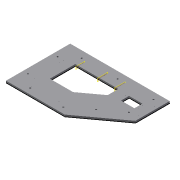
# Autodesk Inventor part: plate
Saved by Autodesk Inventor 2022 (Build 260148000, 148)
## iProperties
Created: 2006-05-17
Part Number: plate
Document SubType Name: Modeling
Designer: dchu
Density: 1 g/cm^3
Material: Generic
Appearance: Default
Author: dchu
Autodesk Inventor part; units mm, degrees
ref_plane "YZ Plane" through (0, 0, 0) normal (1, 0, 0) x (0, 1, 0)
ref_plane "XZ Plane" through (0, 0, 0) normal (0, 1, 0) x (-1, 0, 0)
ref_plane "XY Plane" through (0, 0, 0) normal (0, 0, 1) x (1, 0, 0)
sketch "Sketch1" plane through (0, 0, 0) normal (0, 0, 1) x (1, 0, 0)
  line L0 (1080.9387, 856.8456) -> (-31.0901, 856.8456)
  line L1 (-31.0901, 856.8456) -> (-31.0901, 139.4979)
  line L2 (-31.0901, 139.4979) -> (626.2703, 139.4979)
  line L3 (626.2703, 139.4979) -> (1080.9387, 473.3358)
  line L4 (1080.9387, 473.3358) -> (1080.9387, 856.8456)
  line L5 (963.1788, 520.0847) -> (751.3683, 364.564) construction
  line L6 (195.0188, 687.1378) -> (677.0148, 687.1378)
  line L7 (677.0148, 687.1378) -> (677.0148, 567.5728)
  line L8 (677.0148, 567.5728) -> (453.8217, 403.6944)
  line L9 (453.8217, 403.6944) -> (195.0188, 403.6944)
  line L10 (195.0188, 403.6944) -> (195.0188, 687.1378)
  line L11 (804.0525, 679.6649) -> (953.5087, 679.6649)
  line L12 (953.5087, 679.6649) -> (953.5087, 589.9913)
  line L13 (953.5087, 589.9913) -> (804.0525, 589.9913)
  line L14 (804.0525, 589.9913) -> (804.0525, 679.6649)
  point P0 (175.6092, 779.9153)
  point P1 (575.6092, 779.9153)
  point P2 (975.6092, 781.6554)
  point P3 (545.6092, 203.1178)
  point P4 (175.6092, 203.1178)
  point P5 (25, 660.086)
  point P6 (25, 328.8534)
  dimension "d1" = 400
  dimension "d2" = 400
  dimension "d3" = 370
  constraints: 30 end point, 8 parallel, 4 perpendicular, 2 horizontal, 2 horizontal alignment, 2 vertical alignment
  measures "d1" distance of point (575.609, 779.915) point (175.609, 779.915)
  measures "d2" horizontal distance of point (975.609, 781.655) point (575.609, 779.915)
  measures "d3" distance of point (545.609, 203.118) point (175.609, 203.118)
extrude "Extrusion1" add sketch "Sketch1" along normal blind 20
sketch "Sketch2" plane through (0, 0, 20) normal (0, 0, 1) x (1, 0, 0)
  point P0 (784.2966, 660.4305)
  point P1 (784.2966, 613.0548)
  point P2 (971.9413, 613.0548)
  point P3 (971.9413, 660.4305)
  point P4 (93.4007, 660.4305)
  point P5 (93.4007, 613.0548)
  point P6 (470.1501, 736.9158)
  point P7 (1046.3575, 723.9381)
  point P8 (1046.3575, 539.6556)
  point P9 (470.1501, 230.7876)
  point P10 (163.8777, 230.7876)
  point P11 (106.776, 316.4401)
  point P12 (656.459, 728.2437)
  point P13 (231.1299, 728.2437)
hole "Hole1" at (784.2966, 660.4305, 20) at (784.2966, 613.0548, 20) at (971.9413, 613.0548, 20) at (971.9413, 660.4305, 20) at (93.4007, 660.4305, 20) at (93.4007, 613.0548, 20) at (470.1501, 736.9158, 20) at (1046.3575, 723.9381, 20) at (1046.3575, 539.6556, 20) at (470.1501, 230.7876, 20) at (163.8777, 230.7876, 20) at (106.776, 316.4401, 20) at (231.1299, 728.2437, 20) at (656.459, 728.2437, 20) direction (0, 0, -1) diameter 5 end through all
sketch "Sketch3" plane through (0, 0, 20) normal (0, 0, 1) x (1, 0, 0)
  line L0 (-31.0901, 139.4979) -> (626.2703, 139.4979)
  line L1 (626.2703, 139.4979) -> (1080.9387, 473.3358)
  line L2 (1080.9387, 473.3358) -> (1080.9387, 856.8456)
  line L3 (963.1788, 520.0847) -> (751.3683, 364.564) construction
  point P0 (175.6092, 779.9153)
  point P1 (575.6092, 779.9153)
  point P2 (975.6092, 781.6554)
  point P3 (545.6092, 203.1178)
  point P4 (175.6092, 203.1178)
  point P5 (25, 660.086)
  point P6 (25, 328.8534)
  dimension "d18" = 400
  dimension "d19" = 400
  dimension "d20" = 370
  constraints: 8 end point, 2 horizontal alignment, 2 vertical alignment, 1 parallel
  measures "d18" distance of point (575.609, 779.915) point (175.609, 779.915)
  measures "d19" horizontal distance of point (975.609, 781.655) point (575.609, 779.915)
  measures "d20" distance of point (545.609, 203.118) point (175.609, 203.118)
hole "Hole2" at (25, 328.8534, 20) at (25, 660.086, 20) at (175.6092, 779.9153, 20) at (575.6092, 779.9153, 20) at (975.6092, 781.6554, 20) at (963.1788, 520.0847, 20) at (751.3683, 364.564, 20) at (545.6092, 203.1178, 20) at (175.6092, 203.1178, 20) direction (0, 0, -1) diameter 17.294 end through all
ref_plane "Work Plane1" through (231.1299, 728.2437, 20) normal (1, 0, 0) x (0, 0, -1)
ref_plane "Work Plane2" through (470.1501, 736.9158, -1303.4787) normal (1, 0, 0) x (0, 0, 1)
ref_plane "Work Plane3" through (656.459, 728.2437, 20) normal (1, 0, 0) x (0, 0, -1)
body "Solid1"
